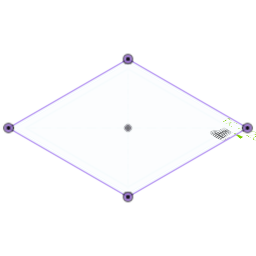
wortuhr (Autodesk Fusion 360 design; units mm, degrees)
Autodesk Fusion 360 part; units mm, degrees
sketch "Skizze2" plane through (0, 0, 0) normal (0, 0, 1) x (1, 0, 0)
  line L0 (97.5, 97.5) -> (-97.5, 97.5)
  line L1 (-97.5, 97.5) -> (-97.5, -97.5)
  line L2 (-97.5, -97.5) -> (97.5, -97.5)
  line L3 (97.5, -97.5) -> (97.5, 97.5)
  line L4 (97.5, 97.5) -> (-97.5, -97.5) construction
  line L5 (-97.5, 97.5) -> (97.5, -97.5) construction
  line L6 (83.5, 83.5) -> (-83.5, 83.5)
  line L7 (-83.5, 83.5) -> (-83.5, -83.5)
  line L8 (-83.5, -83.5) -> (83.5, -83.5)
  line L9 (83.5, -83.5) -> (83.5, 83.5)
  line L10 (83.5, 83.5) -> (-83.5, -83.5) construction
  line L11 (-83.5, 83.5) -> (83.5, -83.5) construction
  dimension "d33" = 195
  dimension "d34" = 195
  dimension "d35" = 167
  dimension "d36" = 167
  constraint horizontal L0
  constraint perpendicular L0 L1
  constraint parallel L0 L2
  constraint parallel L1 L3
  constraint coincident L4 origin
  constraint coincident L5 origin
  constraint horizontal L6
  constraint perpendicular L6 L7
  constraint parallel L6 L8
  constraint parallel L7 L9
  constraint coincident L10 origin
  constraint coincident L11 origin
  measures "d33" distance of L1.end L2.end
  measures "d34" distance of L0.end L1.end
  measures "d35" distance of L7.end L8.end
  measures "d36" distance of L6.end L7.end
sketch "Skizze5" plane through (0, 0, 0) normal (0, 0, 1) x (1, 0, 0)
  line L0 (97.5, -97.5) -> (97.5, 97.5)
  line L1 (97.5, 97.5) -> (-97.5, 97.5)
  line L2 (-97.5, 97.5) -> (-97.5, -97.5)
  line L3 (-97.5, -97.5) -> (97.5, -97.5)
  line L4 (-93.3, 93.3) -> (-93.3, -93.3)
  line L5 (-93.3, -93.3) -> (93.3, -93.3)
  line L6 (93.3, -93.3) -> (93.3, 93.3)
  line L7 (93.3, 93.3) -> (-93.3, 93.3)
extrude "Extrusion2" add sketch "Skizze5" against normal blind 2 contours L4 L5 L6 L7
sketch "Skizze6" plane through (0, 0, 0) normal (0, 0, 1) x (1, 0, 0)
  line L0 (-93.3, -93.3) -> (93.3, -93.3)
  line L1 (-93.3, 93.3) -> (-93.3, -93.3)
  line L2 (-83.5, -80.45) -> (83.5, -80.45)
  line L3 (83.5, -80.45) -> (83.5, -69.45)
  line L4 (83.5, -69.45) -> (-83.5, -69.45)
  line L5 (-83.5, -69.45) -> (-83.5, -80.45)
  line L6 (93.3, -93.3) -> (93.3, 93.3)
  line L7 (-93.3, -93.3) -> (93.3, -93.3)
  line L8 (0, 1.75) -> (0, 22.5)
  dimension "d47" = 167
  dimension "d48" = 11
  dimension "d50" = 9.8
  dimension "d51" = 12.85
  constraint horizontal L2
  constraint vertical L3
  constraint horizontal L4
  constraint vertical L5
  constraint symmetric L3 L5 L8
  measures "d47" distance of L2.start L2.end
  measures "d48" distance of L2.start L4.end
  measures "d50" distance of L3 L6
  measures "d51" distance of L2 L7
extrude "Extrusion3" cut sketch "Skizze6" against normal blind 0.4
pattern_linear "R-Anordnung1" count 10 spacing 16.7 along (0, 1, 0) of "Extrusion3"
sketch "Skizze7" plane through (0, 0, 0) normal (0, 0, 1) x (1, 0, 0)
  line L0 (97.5, -97.5) -> (97.5, 97.5)
  line L1 (97.5, 97.5) -> (-97.5, 97.5)
  line L2 (-97.5, 97.5) -> (-97.5, -97.5)
  line L3 (-97.5, -97.5) -> (97.5, -97.5)
  line L4 (-93.3, 93.3) -> (-93.3, -93.3)
  line L5 (-93.3, -93.3) -> (93.3, -93.3)
  line L6 (93.3, -93.3) -> (93.3, 93.3)
  line L7 (93.3, 93.3) -> (-93.3, 93.3)
extrude "Extrusion4" [rolled back] taper angle 0
sketch "Skizze8" plane through (0, 0, -2) normal (0, 0, 1) x (-1, 0, 0)
  line L0 (-93.3, -93.3) -> (93.3, -93.3)
  line L1 (93.3, -93.3) -> (93.3, 93.3)
  line L2 (93.3, 93.3) -> (-93.3, 93.3)
  line L3 (-93.3, 93.3) -> (-93.3, -93.3)
  line L4 (76.6, 92.1) -> (92.1, 92.1)
  line L5 (92.1, 92.1) -> (92.1, 76.6)
  line L6 (92.1, 76.6) -> (76.6, 76.6)
  line L7 (76.6, 76.6) -> (76.6, 92.1)
  line L8 (93.3, -93.3) -> (93.3, 93.3)
  line L9 (93.3, 93.3) -> (-93.3, 93.3)
  line L10 (84.35, 76.6) -> (84.35, 92.1) construction
  line L11 (81.6, 81.6) -> (87.1, 81.6)
  line L12 (87.1, 81.6) -> (87.1, 87.1)
  line L13 (87.1, 87.1) -> (81.6, 87.1)
  line L14 (81.6, 87.1) -> (81.6, 81.6)
  line L15 (81.6, 81.6) -> (87.1, 87.1) construction
  line L16 (87.1, 81.6) -> (81.6, 87.1) construction
  point P0 (84.35, 84.35)
  point P1 (84.35, 84.35)
  dimension "d74" = 15.5
  dimension "d75" = 15.5
  dimension "d76" = 1.2
  dimension "d77" = 1.2
  dimension "d82" = 5.5
  dimension "d83" = 5.5
  constraint horizontal L4
  constraint vertical L5
  constraint horizontal L6
  constraint vertical L7
  constraint midpoint L6 L10.start
  constraint midpoint L4 L10.end
  constraint midpoint L10 P1
  constraint horizontal L11
  constraint perpendicular L11 L12
  constraint parallel L11 L13
  constraint parallel L12 L14
  constraint coincident L15 P1
  constraint coincident L16 P1
  constraint coincident P1 P0
  measures "d74" distance of L4.start L4.end
  measures "d75" distance of L4.start L6.end
  measures "d76" distance of L5 L8
  measures "d77" distance of L4 L9
  measures "d82" distance of L12.end L13.end
  measures "d83" distance of L11.end L12.end
extrude "Extrusion7" [rolled back] taper angle 0
extrude "Extrusion8" [rolled back] taper angle 0
pattern_linear "R-Anordnung3" [rolled back] u space distance 16.7 v space distance 16.7
extrude "Extrusion6" [rolled back] taper angle 0
sketch "Skizze9" plane through (0, 0, 0) normal (0, 0, 1) x (1, 0, 0)
  line L0 (-93.3, 93.3) -> (-93.3, -93.3)
  line L1 (-93.3, -93.3) -> (93.3, -93.3)
  line L2 (-93.3, -93.3) -> (-92.1, -93.3)
  line L3 (-92.1, 93.4162) -> (-93.3, 93.4162)
  line L4 (-93.3, 93.4162) -> (-93.3, -93.3)
  dimension "d73" = 1.2
  constraint horizontal L2
  constraint horizontal L3
  constraint vertical L4
  constraint coincident L0.end L1.start
  measures "d73" distance of L0.end L2.end
extrude "Extrusion5" [rolled back] taper angle 0
pattern_linear "R-Anordnung2" [rolled back] u space distance 16.7 v space distance 16.7
hidden bodies 1
equation "ledPitch = 16.7 mm" comment "LED-Abstand"
equation "gridCols = 10" comment "LED-Spalten"
equation "gridRows = 10" comment "LED-Reihen"
equation "stripWidth = 11 mm" comment "Strip-Breite + Toleranz"
equation "stripHeightCut = 0.4 mm" comment "Strip-Hoehe an Schneidstelle"
equation "ledHeight = 1.6 mm" comment "LED-Hoehe ueber Strip"
equation "ledSize = 5.5 mm" comment "LED-Kantenlaenge"
equation "frontThk = 2.0 mm" comment "Frontplatten-Dicke"
equation "letterThk = 0.2 mm" comment "Buchstaben-Restwand (1 Layer)"
equation "diffuserSlot = 0.4 mm" comment "Spalt fuer Pauspapier-Diffusor"
equation "gridHeight = 15 mm" comment "Lichtgitter-Hoehe"
equation "gridWall = 1.2 mm" comment "Steg-Dicke Gitter"
equation "carrierThk = 2.0 mm" comment "LED-Traegerplatten-Dicke"
equation "carrierGroove = 0.4 mm" comment "Strip-Rille-Tiefe"
equation "elecDepth = 30 mm" comment "Elektronikraum-Tiefe"
equation "backThk = 2.0 mm" comment "Rueckwand-Dicke"
equation "frameWall = 4 mm" comment "Rahmenwand-Dicke"
equation "wireMargin = 10 mm" comment "Verkabelungsrand umlaufend"
equation "falzDepth = 1.5 mm" comment "Falz-Tiefe Frontplatte/Rahmen"
equation "falzWidth = 2.5 mm" comment "Falz-Breite Frontplatte/Rahmen"
equation "fitTol = 0.2 mm" comment "Allgemeine Passungs-Toleranz"
equation "insertDia = 4.2 mm" comment "Heat-Set Insert Lochdurchmesser"
equation "insertDepth = 5 mm" comment "Heat-Set Insert Lochtiefe"
equation "innerSize = ledPitch * gridCols" comment "Raster-Innenmass"
equation "outerSize = innerSize + 2 * wireMargin + 2 * frameWall" comment "Aussenmass Uhr"
equation "totalDepth = frontThk + diffuserSlot + gridHeight + carrierThk + elecDepth + backThk" comment "Gesamttiefe"
equation "stripPassage = stripHeightCut + fitTol" comment "Aussparung Gitter-Quersteg fuer Strip"
equation "gridCellSize = ledPitch - gridWall" comment "Innere Zellgroesse Gitter"
equation "d33 = outerSize"
equation "d34 = outerSize"
equation "d35 = innerSize"
equation "d36 = innerSize"
equation "d40 = -frameWall - fitTol"
equation "d41 = -carrierThk"
equation "d47 = innerSize"
equation "d48 = stripWidth"
equation "d51 = wireMargin + ( ledPitch - stripWidth ) / 2"
equation "d52 = -carrierGroove"
equation "d54 = gridRows"
equation "d56 = ledPitch"
equation "solderClear = 5 mm" comment "Lötzugang, Pads hängen in der Luft"
equation "d59 = -frameWall - fitTol"
equation "d60 = -carrierThk"
equation "d61 = -gridHeight"
equation "d65 = -gridHeight"
equation "d67 = gridCols"
equation "d68 = gridRows"
equation "d69 = ledPitch"
equation "d70 = ledPitch"
equation "d71 = -gridCellSize"
equation "d73 = gridWall"
equation "d74 = gridCellSize"
equation "d75 = gridCellSize"
equation "d76 = gridWall"
equation "d77 = gridWall"
equation "d78 = -gridHeight + gridWall"
equation "d82 = ledSize"
equation "d83 = ledSize"
equation "d84 = -gridHeight"
equation "d86 = gridRows"
equation "d87 = gridCols"
equation "d88 = ledPitch"
equation "d89 = ledPitch"
named bodies: "LED-Trägerplatte", "Gitter"
